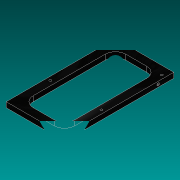
# Autodesk Inventor part: コックピット_2_サブフレーム_1
Saved by Autodesk Inventor 2016 (Build 200138000, 138)
## iProperties
Created: 2016-05-24
Part Number: コックピット_2_サブフレーム_1
Material: アセタール樹脂、黒
Document SubType Name: Modeling
Designer: hiroaki
Density: 1.425 g/cm^3
Appearance: 滑らか - 黒
Mass: 16.9771 g
Surface Area: 78.066 cm^2
Volume: 11.9138 cm^3
Author: hiroaki
Autodesk Inventor part; units mm, degrees
ref_plane "YZ Plane" through (0, 0, 0) normal (1, 0, 0) x (0, 1, 0)
ref_plane "XZ Plane" through (0, 0, 0) normal (0, 1, 0) x (-1, 0, 0)
ref_plane "XY Plane" through (0, 0, 0) normal (0, 0, 1) x (1, 0, 0)
sketch "スケッチ1" plane through (0, 0, 0) normal (0, 0, 1) x (1, 0, 0)
  line L0 (-28, -52.5) -> (28, -52.5) construction
  line L1 (28, -52.5) -> (28, 52.5) construction
  line L2 (28, 52.5) -> (-28, 52.5) construction
  line L3 (-28, 52.5) -> (-28, -52.5) construction
  line L4 (-28, -52.5) -> (28, 52.5) construction
  line L5 (28, -52.5) -> (-28, 52.5) construction
  line L6 (-28, -52.5) -> (-28, 52.5)
  line L7 (-28, 52.5) -> (28, 52.5)
  line L8 (28, 52.5) -> (28, -52.5)
  line L9 (-28, -52.5) -> (28, -52.5)
  line L10 (0, 0) -> (0, 52.5) construction
  line L11 (0, 0) -> (28, 0) construction
  line L12 (-24.5, 44.5) -> (24.5, 44.5) construction
  line L13 (24.5, 44.5) -> (24.5, -13.5) construction
  line L14 (24.5, -13.5) -> (-24.5, -13.5) construction
  line L15 (-24.5, -13.5) -> (-24.5, 44.5) construction
  line L16 (-24.5, 44.5) -> (24.5, -13.5) construction
  line L17 (24.5, 44.5) -> (-24.5, -13.5) construction
  circle A0 centre (-24.5, 44.5) radius 1.04
  circle A1 centre (-24.5, -13.5) radius 1.04
  circle A2 centre (24.5, -13.5) radius 1.04
  circle A3 centre (24.5, 44.5) radius 1.04
  point P0 (0, 15.5)
  point P1 (0, 15.5)
  point P2 (0, 0)
  dimension "d9" = 56
  dimension "d12" = 105
  dimension "d52" = 2.08
  dimension "d53" = 49
  dimension "d54" = 58
  dimension "d55" = 8
  constraints: 36 end point, 8 midpoint, 5 perpendicular, 4 centre point, 4 coincident, 4 parallel, 3 collinear, 3 equal radius, 2 horizontal, 1 symmetric about line, 1 vertical, 1 vertical alignment
  measures "d9" distance of L1.end L2.end
  measures "d12" distance of L0.end L1.end
  measures "d52" diameter of A0
  measures "d53" distance of L12.start L12.end
  measures "d54" distance of L14.end L12.start
  measures "d55" distance between parallel lines of L2 L12
extrude "押し出し1" add sketch "スケッチ1" along normal blind 5
sketch "スケッチ3" plane through (0, 0, 5) normal (0, 0, 1) x (1, 0, 0)
  line L0 (28, 52.5) -> (-28, 52.5) projected
  line L1 (-28, 52.5) -> (-28, -52.5) projected
  line L2 (-20, -44.5) -> (20, -44.5)
  line L3 (20, -44.5) -> (20, 44.5)
  line L4 (20, 44.5) -> (-20, 44.5)
  line L5 (-20, 44.5) -> (-20, -44.5)
  line L6 (-20, -44.5) -> (20, 44.5) construction
  line L7 (20, -44.5) -> (-20, 44.5) construction
  point P0 (-28, 42.1)
  point P1 (0, 0)
  dimension "d47" = 8
  dimension "d48" = 8
  constraints: 12 end point, 2 midpoint, 2 parallel, 1 horizontal, 1 perpendicular
  measures "d47" distance between parallel lines of L1 L5
  measures "d48" distance between parallel lines of L0 L4
extrude "押し出し3" cut sketch "スケッチ3" against normal blind 10
fillet "フィレット1" radius 10 4 edges at (-20, 44.5, 2.5) (20, 44.5, 2.5) (20, -44.5, 2.5) (-20, -44.5, 2.5)
sketch "スケッチ4" plane through (-28, -52.5, 0) normal (-1, 0, 0) x (0, 0, 1)
  line L0 (0, 0) -> (5, 0) projected
  line L1 (0, 105) -> (5, 105) projected
  point P0 (0, 52.5)
  point P1 (2.5, 90)
  point P2 (2.5, 15)
  point P3 (2.5, 105)
  dimension "d73" = 15
  dimension "d74" = 15
  constraints: 2 vertical alignment, 1 midpoint
  measures "d73" distance from line of L1 point (2.5, 90)
  measures "d74" distance from line of L0 point (2.5, 15)
hole "穴1" at (-28, 37.5, 2.5) at (-28, -37.5, 2.5) direction (1, 0, 0) diameter 2.459 depth 2.5 thread size "M3x0.5" class "6H" standard "ISO Metric profile"
mirror "ミラー1" about plane through (0, 0, 0) normal (1, 0, 0) of "穴1"
equation "\"d12\" = d19"
equation "\"d55\" = d69"
equation "\"d47\" = d48"
equation "\"d73\" = d21"
equation "\"d74\" = d22"
equation "\"d19\" = 105"
equation "\"d69\" = 8"
equation "\"d21\" = 15"
equation "\"d22\" = 15"
